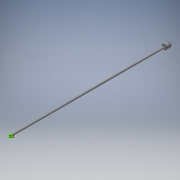
# Autodesk Inventor part: base
Saved by Autodesk Inventor 2018 (Build 220112000, 112)
## iProperties
Created: 2017-12-24
Part Number: base
Material: Generic
Document SubType Name: Modeling
Designer: Hembramone
Density: 1 g/cm^3
Appearance: Default
Author: Hembramone
Autodesk Inventor part; units mm, degrees
ref_plane "YZ Plane" through (0, 0, 0) normal (1, 0, 0) x (0, 1, 0)
ref_plane "XZ Plane" through (0, 0, 0) normal (0, 1, 0) x (-1, 0, 0)
sketch "Sketch1" plane through (0, 0, 0) normal (1, 0, 0) x (0, 1, 0)
  point P0 (0, 0)
sketch "Sketch2" plane through (0, 0, 0) normal (0, 0, 1) x (1, 0, 0)
  circle A0 centre (0, 0) radius 750
  dimension "d0" = 1500
  constraints: 1 centre point, 1 coincident
  measures "d0" diameter of A0
ref_plane "Work Plane1" through (-26382.6859, -30000, -123714.275) normal (0, 0, -1) x (0, 1, 0)
extrude "Extrusion1" add sketch "Sketch2" against normal up to surface (123714.275 mm away)
sketch "Sketch3" plane through (0, 0, -123714.275) normal (0, 0, -1) x (-1, 0, 0)
  circle A0 centre (0, 0) radius 2000
  dimension "d3" = 4000
  constraints: 1 centre point, 1 coincident
  measures "d3" diameter of A0
extrude "Extrusion2" add sketch "Sketch3" along normal blind 4000
fillet "Fillet1" radius 1000 1 edges at (2000, 0, -127714.275)
sketch "Sketch4" plane through (0, 0, -127714.275) normal (0, 0, -1) x (-1, 0, 0)
  circle A0 centre (0, 0) radius 400
  dimension "d7" = 800
  constraints: 1 centre point, 1 coincident
  measures "d7" diameter of A0
extrude "Extrusion3" cut sketch "Sketch4" against normal through all
sketch "Sketch5" plane through (0, 0, 0) normal (0, 0, 1) x (1, 0, 0)
  circle A0 centre (0, 0) radius 400
  circle A1 centre (0, 0) radius 1600
  dimension "d10" = 3200
  constraints: 2 centre point, 1 coincident
  measures "d10" diameter of A1
body "Solid1"
